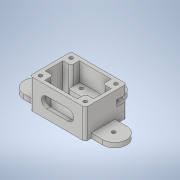
# Autodesk Inventor part: Caixa CG
Saved by Autodesk Inventor 2021 (Build 250183000, 183)
## iProperties
Created: 2021-05-27
Part Number: Caixa CG
Material: Generic
Document SubType Name: Modeling
Designer: hoope
Density: 1 g/cm^3
Appearance: Default
Author: hoope
Autodesk Inventor part; units mm, degrees
ref_plane "YZ Plane" through (0, 0, 0) normal (1, 0, 0) x (0, 1, 0)
ref_plane "XZ Plane" through (0, 0, 0) normal (0, 1, 0) x (-1, 0, 0)
ref_plane "XY Plane" through (0, 0, 0) normal (0, 0, 1) x (1, 0, 0)
sketch "Esboço1" plane through (0, 0, 0) normal (0, 1, 0) x (-1, 0, 0)
  line L0 (0, 0) -> (47, 0)
  line L1 (47, 0) -> (47, 35)
  line L2 (47, 35) -> (0, 35)
  line L3 (0, 35) -> (0, 0)
  dimension "d0" = 47
  dimension "d1" = 35
  constraints: 8 end point, 2 parallel, 1 horizontal, 1 perpendicular
  measures "d0" distance of L2.end L1.end
  measures "d1" distance of L1.end L0.end
extrude "Extrusão1" add sketch "Esboço1" along normal blind 25
shell "Casca1" thickness 3 removed faces 1 at (-15.6667, 25, 23.3333)
sketch "Esboço2" plane through (-47, 0, 35) normal (0, 0, 1) x (1, 0, 0)
  arc A0 (14.5, 17.15) -> (14.5, 7.85) centre (14.5, 12.5) ccw
  line L0 (0, 25) -> (47, 25) projected
  arc A1 (32.5, 7.85) -> (32.5, 17.15) centre (32.5, 12.5) ccw
  line L1 (47, 0) -> (47, 25) projected
  line L2 (14.5, 17.15) -> (32.5, 17.15)
  line L3 (32.5, 7.85) -> (14.5, 7.85)
  line L4 (0, 0) -> (0, 25) projected
  dimension "d5" = 9.3
  dimension "d6" = 12.5
  dimension "d7" = 9.3
  dimension "d8" = 18
  dimension "d9" = 14.5
  constraints: 4 end point, 4 point on circle, 2 centre point, 1 horizontal, 1 parallel
  measures "d5" diameter of A0
  measures "d6" distance from line of L0 A0.centre
  measures "d7" diameter of A1
  measures "d8" distance of A1.centre A0.centre
  measures "d9" distance from line of L1 A1.centre
extrude "Extrusão2" cut sketch "Esboço2" against normal blind 10
sketch "Esboço3" plane through (-44, 3, 3) normal (0, 1, 0) x (1, 0, 0)
  line L0 (41, 0) -> (0, 0) projected
  line L1 (0, 0) -> (7, 0)
  line L2 (7, 0) -> (7, -7)
  line L3 (7, -7) -> (0, -7)
  line L4 (0, -7) -> (0, 0)
  line L5 (41, 0) -> (34, 0)
  line L6 (34, 0) -> (34, -7)
  line L7 (34, -7) -> (41, -7)
  line L8 (41, -7) -> (41, 0)
  line L9 (41, -29) -> (34.3, -29)
  line L10 (34.3, -29) -> (34.3, -22)
  line L11 (34.3, -22) -> (41, -22)
  line L12 (41, -22) -> (41, -29)
  line L13 (41, -29) -> (0, -29) projected
  line L14 (0, -29) -> (6.7, -29)
  line L15 (6.7, -29) -> (6.7, -22)
  line L16 (6.7, -22) -> (0, -22)
  line L17 (0, -22) -> (0, -29)
  point P0 (44, 3)
  dimension "d12" = 7
  dimension "d13" = 7
  dimension "d14" = 7
  dimension "d15" = 7
  dimension "d16" = 6.7
  dimension "d17" = 7
  dimension "d18" = 6.7
  dimension "d19" = 7
  constraints: 32 end point, 8 parallel, 4 horizontal, 4 perpendicular
  measures "d12" distance of L2.end L3.end
  measures "d13" distance of L1.end L2.end
  measures "d14" distance of L7.end L6.end
  measures "d15" distance of L6.end L5.end
  measures "d16" distance of L10.end L11.end
  measures "d17" distance of L9.end L10.end
  measures "d18" distance of L16.end L15.end
  measures "d19" distance of L15.end L14.end
extrude "Extrusão3" add sketch "Esboço3" along normal blind 22
sketch "Esboço4" plane through (-37, 3, 3) normal (0, 1, 0) x (1, 0, 0)
  line L0 (27, 0) -> (27, -7) projected
  line L1 (0, -7) -> (0, 0) projected
  line L2 (0, 0) -> (27, 0) projected
  line L3 (27, 0) -> (0, 0) projected
  line L4 (0.5, 0) -> (26.5, 0)
  line L5 (26.5, 0) -> (26.5, -10)
  line L6 (26.5, -10) -> (0.5, -10)
  line L7 (0.5, -10) -> (0.5, 0)
  line L8 (5.72, -0.65) -> (8.6212, -2.325)
  line L9 (8.6212, -2.325) -> (8.6212, -5.675)
  line L10 (8.6212, -5.675) -> (5.72, -7.35)
  line L11 (5.72, -7.35) -> (2.8188, -5.675)
  line L12 (2.8188, -5.675) -> (2.8188, -2.325)
  line L13 (2.8188, -2.325) -> (5.72, -0.65)
  line L14 (21.28, -0.65) -> (24.1812, -2.325)
  line L15 (24.1812, -2.325) -> (24.1812, -5.675)
  line L16 (24.1812, -5.675) -> (21.28, -7.35)
  line L17 (21.28, -7.35) -> (18.3788, -5.675)
  line L18 (18.3788, -5.675) -> (18.3788, -2.325)
  line L19 (18.3788, -2.325) -> (21.28, -0.65)
  point P0 (37, 3)
  point P1 (5.72, -4)
  point P2 (21.28, -4)
  dimension "d33" = 26
  dimension "d34" = 10
  dimension "d35" = 0.5
  constraints: 32 end point, 2 parallel, 1 horizontal, 1 perpendicular, 1 point on line, 26 other
  measures "d33" distance between parallel lines of L5 L7
  measures "d34" distance between parallel lines of L4 L6
  measures "d35" distance between parallel lines of L0 L5
fillet "Arredondamento1" radius 2 4 edges at (-47, 12.5, 35) (0, 12.5, 35) (0, 12.5, 0) (-47, 12.5, 0)
fillet "Arredondamento2" radius 2 4 edges at (-37, 14, 10) (-10, 14, 10) (-37.3, 14, 25) (-9.7, 14, 25)
sketch "Esboço35" plane through (0, 0, 33) normal (1, 0, 0) x (0, 0, -1)
  line L0 (31, 0) -> (0, 0) projected
  line L1 (3, 0) -> (23, 0)
  line L2 (23, 0) -> (23, 4)
  line L3 (23, 4) -> (3, 4)
  line L4 (3, 4) -> (3, 0)
  line L5 (-2, 25) -> (-2, 0) projected
  point P0 (33, 0)
  dimension "d160" = 20
  dimension "d161" = 4
  dimension "d162" = 5
  constraints: 8 end point, 2 parallel, 1 horizontal, 1 perpendicular, 1 point on line
  measures "d160" distance of L3.end L2.end
  measures "d161" distance of L2.end L1.end
  measures "d162" distance between parallel lines of L5 L4
extrude "Extrusão26" add sketch "Esboço35" along normal blind 20
sketch "Esboço36" plane through (-2, 0, 0) normal (0, 0, -1) x (-1, 0, 0)
  line L0 (11.5, 0) -> (31.5, 0)
  line L1 (31.5, 0) -> (31.5, 4)
  line L2 (31.5, 4) -> (11.5, 4)
  line L3 (11.5, 4) -> (11.5, 0)
  line L4 (-2, 25) -> (-2, 0) projected
  dimension "d165" = 20
  dimension "d166" = 4
  dimension "d167" = 13.5
  constraints: 8 end point, 2 parallel, 1 horizontal, 1 perpendicular
  measures "d165" distance of L2.end L1.end
  measures "d166" distance of L1.end L0.end
  measures "d167" distance between parallel lines of L4 L3
extrude "Extrusão27" add sketch "Esboço36" along normal blind 20
sketch "Esboço37" plane through (-47, 0, 2) normal (-1, 0, 0) x (0, 0, 1)
  line L0 (8, 4) -> (8, 0) projected
  line L1 (8, 4) -> (28, 4) projected
  line L2 (8, 0) -> (28, 0)
  line L3 (28, 0) -> (28, 4)
  line L4 (28, 4) -> (8, 4)
  line L5 (8, 4) -> (8, 0)
  point P0 (-2, 0)
  constraints: 8 end point, 2 parallel, 1 horizontal, 1 perpendicular
extrude "Extrusão28" add sketch "Esboço37" along normal blind 20
fillet "Arredondamento9" radius 10 6 edges at (-67, 2, 30) (-67, 2, 10) (-33.5, 2, -20) (-13.5, 2, -20) (20, 2, 10) (20, 2, 30)
sketch "Esboço38" plane through (-47, 4, 30) normal (0, 1, 0) x (1, 0, 0)
  circle A0 centre (-9, 10) radius 1.5
  circle A1 centre (23.5, 39) radius 1.5
  circle A2 centre (56, 10) radius 1.5
  line L0 (0, 20) -> (-10, 20) projected
  line L1 (0, 28) -> (0, -3) projected
  line L2 (13.5, 30) -> (13.5, 40) projected
  line L3 (45, 30) -> (2, 30) projected
  line L4 (47, 20) -> (57, 20) projected
  line L5 (47, -3) -> (47, 28) projected
  point P0 (47, 30)
  dimension "d173" = 3
  dimension "d174" = 3
  dimension "d175" = 3
  dimension "d176" = 10
  dimension "d177" = 9
  dimension "d178" = 10
  dimension "d179" = 9
  dimension "d180" = 10
  dimension "d181" = 9
  constraints: 3 centre point
  measures "d173" diameter of A0
  measures "d174" diameter of A1
  measures "d175" diameter of A2
  measures "d176" distance from line of L0 A0.centre
  measures "d177" distance from line of L1 A0.centre
  measures "d178" distance from line of L2 A1.centre
  measures "d179" distance from line of L3 A1.centre
  measures "d180" distance from line of L4 A2.centre
  measures "d181" distance from line of L5 A2.centre
extrude "Extrusão29" cut sketch "Esboço38" against normal blind 20
sketch "Esboço40" plane through (-47, 0, 33) normal (-1, 0, 0) x (0, 0, 1)
  line L0 (-33, 0) -> (-33, 25) projected
  line L1 (-33, 17.5) -> (-24.5, 17.5)
  line L2 (-24.5, 17.5) -> (-24.5, 12.5)
  line L3 (-24.5, 12.5) -> (-33, 12.5)
  line L4 (-33, 12.5) -> (-33, 17.5)
  line L5 (-31, 25) -> (0, 25) projected
  dimension "d222" = 8.5
  dimension "d223" = 5
  dimension "d242" = 7.5
  constraints: 8 end point, 2 parallel, 1 horizontal, 1 perpendicular, 1 point on line
  measures "d222" distance of L2.end L3.end
  measures "d223" distance of L1.end L2.end
  measures "d242" distance between parallel lines of L1 L5
extrude "Extrusão32" cut sketch "Esboço40" against normal blind 8.5
sketch "Esboço42" plane through (0, 25, 0) normal (0, 1, 0) x (1, 0, 0)
  circle A0 centre (-4.5, -4.5) radius 1.505
  line L0 (0, -33) -> (0, -2) projected
  line L1 (-2, 0) -> (-45, 0) projected
  circle A1 centre (-4.5, -30.5) radius 1.505
  circle A2 centre (-42.5, -4.5) radius 1.505
  circle A3 centre (-42.5, -30.5) radius 1.505
  point P0 (0, 0)
  dimension "d226" = 3.01
  dimension "d227" = 4.5
  dimension "d228" = 4.5
  dimension "d231" = 26
  dimension "d234" = 38
  constraints: 4 centre point, 1 horizontal, 1 vertical, 6 other
  measures "d226" diameter of A0
  measures "d227" distance from line of L0 A0.centre
  measures "d228" distance from line of L1 A0.centre
  measures "d231" distance of A0.centre A1.centre
  measures "d234" distance of A0.centre A2.centre
extrude "Extrusão33" cut sketch "Esboço42" against normal blind 20
sketch "Esboço44" plane through (-2, 25, 0) normal (0, 0, -1) x (-1, 0, 0)
  line L0 (-2, -25) -> (-2, 0) projected
  line L1 (-2, -7.5) -> (6.5, -7.5)
  line L2 (6.5, -7.5) -> (6.5, -12.5)
  line L3 (6.5, -12.5) -> (-2, -12.5)
  line L4 (-2, -12.5) -> (-2, -7.5)
  line L5 (0, 0) -> (43, 0) projected
  point P0 (-2, -12.5)
  dimension "d239" = 8.5
  dimension "d240" = 5
  dimension "d241" = 7.5
  constraints: 8 end point, 2 parallel, 1 horizontal, 1 perpendicular, 1 point on line
  measures "d239" distance of L2.end L3.end
  measures "d240" distance of L1.end L2.end
  measures "d241" distance between parallel lines of L5 L1
extrude "Extrusão34" cut sketch "Esboço44" against normal blind 8.5
extrude "Extrusão35" add sketch "Esboço4" along normal blind 4.5
sketch "Esboço46" plane through (-37, 7.5, 3) normal (0, 1, 0) x (1, 0, 0)
  line L0 (0.5, 0) -> (0.5, -10) projected
  line L1 (26.5, 0) -> (26.5, -10) projected
  line L2 (0.5, 0) -> (26.5, 0)
  line L3 (26.5, 0) -> (26.5, -10)
  line L4 (26.5, -10) -> (0.5, -10)
  line L5 (0.5, -10) -> (0.5, 0)
  point P0 (37, 3)
  constraints: 8 end point, 2 parallel, 1 horizontal, 1 perpendicular
extrude "Extrusão36" add sketch "Esboço46" along normal blind 2
sketch "Esboço47" plane through (-37, 9.5, 3) normal (0, 1, 0) x (1, 0, 0)
  circle A0 centre (5.72, -4) radius 1.505
  circle A1 centre (21.28, -4) radius 1.505
  point P0 (37, 3)
  dimension "d251" = 3.01
  dimension "d252" = 3.01
  constraints: 2 centre point
  measures "d251" diameter of A0
  measures "d252" diameter of A1
extrude "Extrusão37" cut sketch "Esboço47" against normal blind 3.01
chamfer "Chanfro5" distance 1.5 angle 45 2 edges at (-36.5, 6.25, 13) (-10.5, 6.25, 13)
